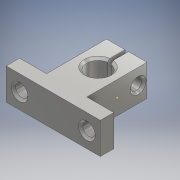
# Autodesk Inventor part: SK10
Saved by Autodesk Inventor 2016 (Build 200138000, 138)
## iProperties
Created: 2016-10-13
Part Number: SK10
Material: Типовые
Document SubType Name: Modeling
Designer: skhalipa
Density: 1 g/cm^3
Appearance: Алюминий — полированный
Author: skhalipa
Autodesk Inventor part; units mm, degrees
ref_plane "YZ Plane" through (0, 0, 0) normal (1, 0, 0) x (0, 1, 0)
ref_plane "XZ Plane" through (0, 0, 0) normal (0, 1, 0) x (-1, 0, 0)
ref_plane "XY Plane" through (0, 0, 0) normal (0, 0, 1) x (1, 0, 0)
sketch "Эскиз1" plane through (0, 0, 0) normal (0, 0, 1) x (1, 0, 0)
  line L0 (-9, 13.4) -> (9, 13.4)
  line L1 (21, -19.4) -> (-21, -19.4)
  line L2 (-21, -19.4) -> (-21, -13.4)
  line L3 (-9, 13.4) -> (-9, -13.4)
  line L4 (9, 13.4) -> (9, -13.4)
  line L5 (21, -19.4) -> (21, -13.4)
  line L6 (-21, -13.4) -> (-9, -13.4)
  line L7 (9, -13.4) -> (21, -13.4)
  point P0 (0, 0)
  point P1 (-9, 0)
  point P2 (0, -19.4)
  dimension "d0" = 42
  dimension "d2" = 18
  dimension "d3" = 9
  dimension "d6" = 6
  dimension "d7" = 32.8
  constraints: 16 end point, 4 horizontal alignment, 3 vertical alignment, 2 midpoint, 2 perpendicular, 1 horizontal, 1 parallel, 1 vertical
  measures "d0" distance of L1.start L1.end
  measures "d2" distance between parallel lines of L4 L3
  measures "d3" distance from line of point (0, 0) L3
  measures "d6" distance of L1.end L2.end
  measures "d7" distance between parallel lines of L1 L0
extrude "Выдавливание1" add sketch "Эскиз1" along normal mid plane 14
sketch "Эскиз3" plane through (0, 0, 7) normal (0, 0, 1) x (1, 0, 0)
  line L0 (-21, -19.4) -> (21, -19.4) projected
  point P0 (0, 0)
  point P1 (0, 0.6)
  dimension "d12" = 20
  constraints: 1 vertical alignment
  measures "d12" distance from line of L0 point (0, 0.6)
hole "Отверстие1" at (0, 0.6, 7) direction (0, 0, -1) diameter 10.2 end through all
sketch "Эскиз4" plane through (0, 0, 7) normal (0, 0, 1) x (1, 0, 0)
  line L0 (-9, 13.4) -> (9, 13.4) projected
  line L1 (-0.75, 13.4) -> (-0.75, 5.6446)
  circle A0 centre (0, 0.6) radius 5.1 projected
  line L2 (0.75, 13.4) -> (0.75, 5.6446)
  point P0 (0, 0)
  dimension "d20" = 1.5
  dimension "d21" = 0.75
  constraints: 4 end point, 2 point on circle, 2 point on line, 1 parallel, 1 perpendicular
  measures "d20" distance between parallel lines of L2 L1
  measures "d21" distance from line of point (0, 0) L1
extrude "Выдавливание2" cut sketch "Эскиз4" against normal blind 14 contours L0 L2 A0 L1
sketch "Эскиз6" plane through (9, -13.4, 7) normal (0, 1, 0) x (1, 0, 0)
  line L0 (12, 14) -> (12, 0) projected
  line L1 (0, 14) -> (12, 14) projected
  point P0 (-9, 7)
  point P1 (6, 7)
  point P2 (12, 7)
  point P3 (6, 14)
  constraints: 2 midpoint, 1 horizontal alignment, 1 vertical alignment
hole "Отверстие3" at (15, -13.4, 0) direction (0, -1, 0) diameter 5.5 end through all
sketch "Эскиз7" plane through (-21, -13.4, 7) normal (0, 1, 0) x (1, 0, 0)
  line L0 (0, 14) -> (12, 14) projected
  line L1 (0, 0) -> (0, 14) projected
  point P0 (21, 7)
  point P1 (6, 7)
  point P2 (6, 14)
  point P3 (0, 7)
  constraints: 2 midpoint, 1 horizontal alignment, 1 vertical alignment
hole "Отверстие4" at (-15, -13.4, 0) direction (0, -1, 0) diameter 5.5 end through all
sketch "Эскиз8" plane through (9, -13.4, 7) normal (1, 0, 0) x (0, 0, -1)
  line L0 (14, 26.8) -> (0, 26.8) projected
  point P0 (7, 13.4)
  point P1 (7, 22.95)
  point P2 (7, 26.8)
  dimension "d50" = 3.85
  constraints: 1 midpoint, 1 vertical alignment
  measures "d50" distance from line of L0 point (7, 22.95)
sketch "Эскиз9" plane through (9, -13.4, 7) normal (1, 0, 0) x (0, 0, -1)
  point P0 (7, 13.4)
hole "Отверстие5" at (9, 9.55, 0) direction (-1, 0, 0) diameter 4.1 end through all
thread "Резьба2" size "M4.5x0.75" class "6H" standard "ANSI Metric M Profile" full length
sketch "Эскиз10" plane through (9, -13.4, 7) normal (1, 0, 0) x (0, 0, -1)
  circle A0 centre (7, 22.95) radius 2.5
  line L0 (14, 26.8) -> (0, 26.8) projected
  point P0 (7, 13.4)
  point P1 (7, 26.8)
  dimension "d60" = 5
  dimension "d61" = 3.85
  constraints: 1 centre point, 1 midpoint, 1 vertical alignment
  measures "d60" diameter of A0
  measures "d61" distance from line of L0 A0.centre
extrude "Выдавливание3" cut sketch "Эскиз10" against normal blind 5
chamfer "Фаска1" distance 1 angle 45 10 edges at (-5.0861, 0.224, 7) (5.0861, 0.224, 7) (-9, 9.55, 2.05) (-15, -19.4, -2.75) (15, -19.4, -2.75) (-5.0861, 0.224, -7) (5.0861, 0.224, -7) (15, -13.4, -2.75) (-15, -13.4, -2.75) (9, 9.55, 2.5)
